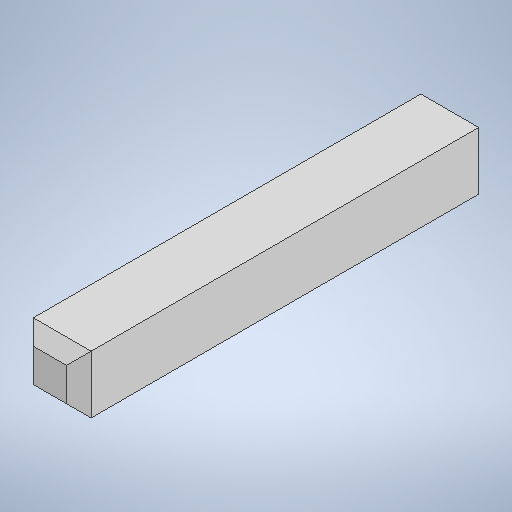
# Autodesk Inventor part: Klin_do_łączenia_34mm
Saved by Autodesk Inventor 2025 (Build 290162000, 162)
## iProperties
Created: 2025-07-30
Part Number: Klin_do_łączenia_34mm
Material: Ogólny
Document SubType Name: Modeling
Designer: ThePi
Density: 1 g/cm^3
Appearance: Domyślna
Author: ThePi
Autodesk Inventor part; units mm, degrees
ref_plane "YZ Plane" through (0, 0, 0) normal (1, 0, 0) x (0, 1, 0)
ref_plane "XZ Plane" through (0, 0, 0) normal (0, 1, 0) x (-1, 0, 0)
ref_plane "XY Plane" through (0, 0, 0) normal (0, 0, 1) x (1, 0, 0)
sketch "Szkic1" plane through (0, 0, 0) normal (0, 0, 1) x (1, 0, 0)
  line L0 (0, 0) -> (-4.5, 0)
  line L1 (-4.5, 0) -> (-4.5, 4.5)
  line L2 (-4.5, 4.5) -> (0, 4.5)
  line L3 (0, 4.5) -> (0, 0)
  line L4 (0, 0) -> (-4.7, 0)
  line L5 (-4.7, 0) -> (-4.7, 4.7)
  line L6 (-4.7, 4.7) -> (0, 4.7)
  line L7 (0, 4.7) -> (0, 0)
  dimension "d0" = 4.5
  dimension "d1" = 4.5
  dimension "d7" = 4.7
  dimension "d8" = 4.7
  constraints: 16 end point, 4 perpendicular, 1 collinear, 1 horizontal, 1 point on line, 1 vertical
  measures "d0" distance of L0.start L0.end
  measures "d1" distance of L0.end L1.end
  measures "d7" distance of L0.start L4.end
  measures "d8" distance of L4.end L5.end
extrude "Wyciągnięcie proste2" add sketch "Szkic1" along normal blind 33.5
chamfer "Faza2" distance 1 angle 45 8 edges at (-4.7, 2.35, 0) (-2.25, 0, 0) (0, 2.25, 0) (-2.35, 4.7, 0) (0, 2.25, 33.5) (-2.25, 0, 33.5) (-4.7, 2.35, 33.5) (-2.35, 4.7, 33.5)
